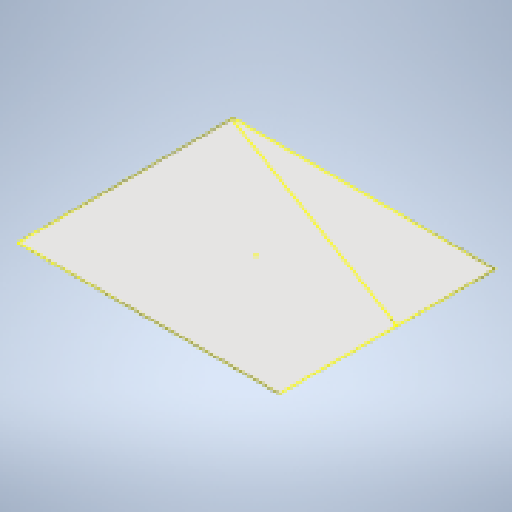
# Autodesk Inventor part: side sheet
Saved by Autodesk Inventor 2025.2 (Build 292293000, 293)
## iProperties
Created: 2025-05-26
Part Number: side sheet
Material: Generic
Document SubType Name: Sheet Metal
Designer: abdal
Density: 1 g/cm^3
Sheet Metal Rule: Default_mm
Appearance: Default
Author: abdal
Autodesk Inventor part; units mm, degrees
ref_plane "YZ Plane" through (0, 0, 0) normal (1, 0, 0) x (0, 1, 0)
ref_plane "XZ Plane" through (0, 0, 0) normal (0, 1, 0) x (-1, 0, 0)
ref_plane "XY Plane" through (0, 0, 0) normal (0, 0, 1) x (1, 0, 0)
sketch "Sketch1" plane through (0, 0, 0) normal (0, 1, 0) x (-1, 0, 0)
  line L0 (473.5, 390) -> (-473.5, 390)
  line L1 (-473.5, 390) -> (-473.5, -390)
  line L2 (-473.5, -390) -> (473.5, -390)
  line L3 (473.5, -390) -> (473.5, 390)
  line L4 (473.5, 390) -> (-473.5, -390) construction
  line L5 (-473.5, 390) -> (473.5, -390) construction
  point P0 (0, 0)
  dimension "d0" = 780
  dimension "d1" = 947
  measures "d0" distance of L0.end L1.end
  measures "d1" distance of L1.end L2.end
extrude "Plate1" add sketch "Sketch1" along normal blind 2
sketch "Sketch2" plane through (0, 2, 0) normal (0, 1, 0) x (1, 0, 0)
  line L0 (-476.5, 385.4593) -> (443.5, 46.5119) projected
  line L1 (449.5, 40) -> (467.5, 40) projected
  arc A0 (473.5, 34) -> (467.5, 40) centre (467.5, 34) ccw projected
  line L2 (449.5, 40) -> (443.5, 46.5119)
  line L3 (473.5, -390) -> (-473.5, -390) projected
  line L4 (473.5, 390) -> (473.5, -390) projected
  line L5 (-473.5, 390) -> (473.5, 390) projected
  line L6 (-473.5, -390) -> (-473.5, 390) projected
  line L7 (443.5, 46.5119) -> (473.5, 35.4593)
  point P0 (0, 0)
  point P1 (-473.5, 384.354)
  point P2 (461.1753, 40)
  point P3 (473.3009, 35.5326)
  constraints: 4 end point, 1 collinear, 1 point on line
extrude "Extrusion1" cut sketch "Sketch2" against normal blind 10 contours L6 L5 L4 L7 A0 L1 L0
equation "\"d2\" = Thickness"
equation "\"BendRadius\" = Thickness"
equation "\"BendReliefWidth\" = Thickness"
equation "\"BendReliefDepth\" = 0.5 * Thickness"
equation "\"CornerReliefSize\" = 4 * Thickness"
equation "\"MinimumRemnant\" = 2 * Thickness"
equation "\"TransitionRadius\" = BendRadius"
equation "\"JacobiRadiusSize\" = BendRadius"
equation "\"GapSize\" = Thickness"
equation "\"Thickness\" = 2"
body "Solid1"
